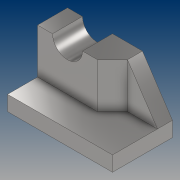
# Autodesk Inventor part: 28
Saved by Autodesk Inventor 2020.2 (Build 242310000, 310)
## iProperties
Created: 2020-09-17
Part Number: 28
Material: 鋼、碳鋼
Document SubType Name: Modeling
Designer: user
Density: 7.85 g/cm^3
Appearance: 半拋光
Mass: 442.413 g
Surface Area: 121.99 cm^2
Volume: 56.3584 cm^3
Author: user
Autodesk Inventor part; units mm, degrees
ref_plane "YZ Plane" through (0, 0, 0) normal (1, 0, 0) x (0, 1, 0)
ref_plane "XZ Plane" through (0, 0, 0) normal (0, 1, 0) x (-1, 0, 0)
ref_plane "XY Plane" through (0, 0, 0) normal (0, 0, 1) x (1, 0, 0)
sketch "草圖1" plane through (0, 0, 0) normal (0, 1, 0) x (-1, 0, 0)
  line L0 (0, 0) -> (-70, 0)
  line L1 (-70, 0) -> (-70, 40)
  line L2 (-70, 40) -> (0, 40)
  line L3 (0, 40) -> (0, 0)
  dimension "d0" = 70
  dimension "d1" = 40
  constraints: 8 end point, 2 parallel, 1 horizontal, 1 perpendicular
  measures "d0" distance of L1.end L2.end
  measures "d1" distance of L2.end L0.start
extrude "擠出1" add sketch "草圖1" along normal blind 10
sketch "草圖2" plane through (0, 10, 0) normal (0, 1, 0) x (1, 0, 0)
  line L0 (0, -40) -> (0, 0) projected
  line L1 (0, 0) -> (70, 0) projected
  line L2 (70, 0) -> (70, -40) projected
  line L3 (70, -40) -> (0, -40) projected
  line L4 (0, 0) -> (70, 0)
  line L5 (70, 0) -> (70, -20)
  line L6 (70, -20) -> (0, -20)
  line L7 (0, -20) -> (0, 0)
  line L8 (70, -40) -> (70, 0) projected
  line L9 (40, -20) -> (50, -10)
  line L10 (50, -10) -> (70, -10)
  point P0 (0, -20)
  dimension "d4" = 20
  dimension "d5" = 10
  dimension "d6" = 20
  dimension "d7" = 30
  constraints: 12 end point, 2 horizontal, 2 parallel, 2 point on line, 1 collinear, 1 perpendicular
  measures "d4" distance between parallel lines of L1 L6
  measures "d5" distance between parallel lines of L1 L10
  measures "d6" distance of L9.end L10.end
  measures "d7" distance from line of L9.start L2
extrude "擠出2" add sketch "草圖2" along normal blind 30 contours L0 L1 L2 L10 L9 L6
sketch "草圖3" plane through (50, 10, 10) normal (0, 0, 1) x (1, 0, 0)
  line L0 (0, 30) -> (0, 0) projected
  line L1 (0, 0) -> (20, 0) projected
  line L2 (20, 0) -> (20, -10) projected
  line L3 (20, -10) -> (-50, -10) projected
  line L4 (-50, -10) -> (-50, 30) projected
  line L5 (-50, 30) -> (0, 30) projected
  line L6 (0, 30) -> (20, 30) projected
  line L7 (20, 30) -> (20, 0) projected
  line L8 (0, 30) -> (20, 30) projected
  line L9 (20, 0) -> (0, 0) projected
  line L10 (0, 30) -> (20, 0)
  constraints: 2 end point
extrude "擠出3" cut sketch "草圖3" against normal blind 10 contours L6 L7 L10
sketch "草圖4" plane through (0, 10, 20) normal (0, 0, 1) x (1, 0, 0)
  line L0 (0, -10) -> (0, 0) projected
  line L1 (0, 0) -> (0, 30) projected
  line L2 (0, 30) -> (40, 30) projected
  line L3 (40, 30) -> (40, 0) projected
  line L4 (40, 0) -> (70, 0) projected
  line L5 (70, 0) -> (70, -10) projected
  line L6 (70, -10) -> (0, -10) projected
  line L7 (0, 0) -> (40, 0) projected
  line L8 (0, 30) -> (40, 30) projected
  circle A0 centre (20, 30) radius 10
  dimension "d12" = 20
  constraints: 1 centre point, 1 midpoint
  measures "d12" diameter of A0
extrude "擠出4" cut sketch "草圖4" against normal blind 46 contours A0 L2 | L2 A0
